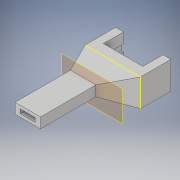
# Autodesk Inventor part: tilt_pillar
Saved by Autodesk Inventor 2018 (Build 220112000, 112)
## iProperties
Created: 2018-04-15
Part Number: tilt_pillar
Material: Generic
Document SubType Name: Modeling
Designer: scwu
Density: 1 g/cm^3
Appearance: Default
Author: scwu
Autodesk Inventor part; units mm, degrees
note: some values were not read from the file. Chosen so that the rebuilt part matches the saved one: second side of "Extrusion5".
ref_plane "YZ Plane" through (0, 0, 0) normal (1, 0, 0) x (0, 1, 0)
ref_plane "XZ Plane" through (0, 0, 0) normal (0, 1, 0) x (-1, 0, 0)
ref_plane "XY Plane" through (0, 0, 0) normal (0, 0, 1) x (1, 0, 0)
sketch "Sketch1" plane through (0, 0, 0) normal (0, 1, 0) x (-1, 0, 0)
  line L0 (-4.4, 0) -> (4.4, 0) construction
  line L1 (0, 0) -> (0, -12) construction
  line L2 (2.65, -12) -> (-2.65, -12) construction
  line L3 (2.65, -12) -> (4.4, 0)
  line L4 (-2.65, -12) -> (-4.4, 0)
  line L5 (0, -12) -> (0, -15.5) construction
  line L6 (0, -15.5) -> (-4, -15.5) construction
  line L7 (0, -15.5) -> (4, -15.5) construction
  line L8 (0, -15.5) -> (4, -15.5) construction
  line L9 (2.65, -12) -> (2.1396, -15.5)
  line L10 (-2.65, -12) -> (-2.1396, -15.5)
  line L11 (2.1396, -15.5) -> (-2.1396, -15.5)
  line L12 (-7.4, 0) -> (12.6, 0) construction
  line L13 (4.4, 0) -> (-4.4, 0)
  dimension "d0" = 8.8
  dimension "d1" = 12
  dimension "d2" = 5.3
  dimension "d3" = 3.5
  dimension "d4" = 4
  dimension "d5" = 4
  dimension "d7" = 3
  constraints: 28 end point, 7 horizontal, 4 collinear, 2 point on line, 2 symmetric about line, 1 midpoint, 1 perpendicular, 1 vertical
  measures "d0" distance of L0.start L0.end
  measures "d1" distance of L1.end L1.start
  measures "d2" distance of L2.start L2.end
  measures "d3" distance of L1.end L5.end
  measures "d4" distance of L5.end L6.end
  measures "d5" distance of L5.end L7.end
  measures "d7" distance of L0.start L12.start
sketch "Sketch2" plane through (0, 0, 0) normal (0, 1, 0) x (-1, 0, 0)
  line L0 (7.4, -46.26) -> (-7.4, -46.26)
  line L1 (-7.4, -46.26) -> (-7.4, 0)
  line L2 (-7.4, 0) -> (7.4, 0)
  line L3 (7.4, 0) -> (7.4, -46.26)
  line L4 (0, 0) -> (0, 4) construction
  line L5 (0, 0) -> (0, -46.26) construction
  dimension "d18" = 4
  dimension "d19" = 50.26
  dimension "d20" = 14.8
  constraints: 12 end point, 2 midpoint, 2 parallel, 2 vertical, 1 horizontal, 1 perpendicular
  measures "d18" distance of L4.start L4.end
  measures "d19" distance of L4.end L5.end
  measures "d20" distance of L1.end L2.end
extrude "Extrusion1" add sketch "Sketch2" along normal mid plane 6
extrude "Extrusion2" cut sketch "Sketch1" along normal mid plane 2.4
sketch "Sketch3" plane through (0, 0, 0) normal (0, 1, 0) x (-1, 0, 0)
  line L0 (0, 0) -> (0, 4) construction
  line L1 (0, 0) -> (0, -46.26) construction
  dimension "d15" = 4
  dimension "d17" = 50.26
  constraints: 4 end point, 2 vertical
  measures "d15" distance of L0.start L0.end
  measures "d17" distance of L0.end L1.end
sketch "Sketch4" plane through (7.4, 3, -46.26) normal (0, 0, -1) x (-1, 0, 0)
  line L0 (-13.95, 5) -> (18.25, 5)
  line L1 (18.25, 5) -> (18.25, -11)
  line L2 (18.25, -11) -> (-13.95, -11)
  line L3 (-13.95, -11) -> (-13.95, 5)
  line L4 (-9.35, 3.1) -> (13.65, 3.1)
  line L5 (13.65, 3.1) -> (13.65, -9.1)
  line L6 (13.65, -9.1) -> (-9.35, -9.1)
  line L7 (-9.35, -9.1) -> (-9.35, 3.1)
  line L8 (2.15, 5) -> (2.15, -11) construction
  line L9 (18.25, -3) -> (-13.95, -3) construction
  line L10 (-9.35, 3.1) -> (-9.35, 5)
  line L11 (13.65, 3.1) -> (13.65, 5)
  line L12 (13.65, -9.1) -> (13.65, -11)
  line L13 (-9.35, -9.1) -> (-9.35, -11)
  circle A0 centre (16.15, -3) radius 1
  circle A1 centre (-11.85, -3) radius 1
  point P0 (7.4, -3)
  point P1 (2.15, -3)
  dimension "d21" = 32.2
  dimension "d22" = 16
  dimension "d23" = 23
  dimension "d24" = 12.2
  dimension "d25" = 2.5
  dimension "d26" = 2
  dimension "d27" = 2.5
  dimension "d28" = 2
  dimension "d43" = 5.25
  constraints: 28 end point, 9 point on line, 5 midpoint, 5 parallel, 2 centre point, 2 coincident, 2 horizontal, 2 perpendicular, 1 horizontal alignment, 2 other
  measures "d21" distance of L1.end L2.end
  measures "d22" distance of L0.end L1.end
  measures "d23" distance of L5.end L6.end
  measures "d24" distance of L4.end L5.end
  measures "d25" distance from line of L5 point (16.15, -3)
  measures "d26" diameter of A0
  measures "d27" distance from line of L7 point (-11.85, -3)
  measures "d28" diameter of A1
  measures "d43" distance of point (7.4, -3) point (2.15, -3)
extrude "Extrusion3" add sketch "Sketch4" along normal blind 15.72 and the other way blind 2 contours L0 L10 L7 L13 L2 L3 | L0 L1 L2 L12 L5 L11
extrude "Extrusion4" add sketch "Sketch4" along normal blind 4 and the other way blind 2 contours L0 L11 L4 L10 | L13 L6 L12 L2
extrude "Extrusion5" add sketch "Sketch4" against normal blind 2 contours A0 | A1
extrude "Extrusion6" add sketch "Sketch4" against normal blind 2 contours L4 L5 L6 L7
sketch "Sketch5" plane through (-10.85, -8, -61.98) normal (-1, 0, 0) x (0, 0, 1)
  line L0 (15.72, 1.9) -> (15.72, 14.1) projected
  line L1 (15.72, 8) -> (6.72, 8) construction
  line L2 (15.72, 6) -> (6.72, 6)
  line L3 (6.72, 6) -> (6.72, 10)
  line L4 (6.72, 10) -> (15.72, 10)
  line L5 (15.72, 10) -> (15.72, 6)
  line L6 (15.72, 6) -> (6.72, 10) construction
  line L7 (6.72, 6) -> (15.72, 10) construction
  point P0 (61.98, 8)
  point P1 (11.22, 8)
  dimension "d44" = 9
  dimension "d45" = 4
  constraints: 14 end point, 4 midpoint, 2 horizontal, 2 parallel, 1 collinear, 1 perpendicular
  measures "d44" distance of L1.start L1.end
  measures "d45" distance of L2.end L3.end
extrude "Extrusion7" cut sketch "Sketch5" against normal blind 6
sketch "Sketch6" plane through (-6.25, -8, -61.98) normal (1, 0, 0) x (0, 0, -1)
  line L0 (-15.72, 10) -> (-6.72, 10) projected
  line L1 (0, 0) -> (0, 16) projected
  line L2 (-6.72, 10) -> (0, 10)
  line L3 (0, 10) -> (0, 6)
  line L4 (0, 6) -> (-6.72, 6)
  line L5 (-6.72, 6) -> (-6.72, 10)
  point P0 (-61.98, 8)
  dimension "d48" = 4
  constraints: 8 end point, 2 parallel, 1 horizontal, 1 perpendicular, 1 point on line
  measures "d48" distance of L2.end L3.end
extrude "Extrusion8" cut sketch "Sketch6" against normal blind 1
ref_plane "Work Plane1" through (7.4, 3, -32.26) normal (0, 0, 1) x (1, 0, 0)
sketch "Sketch7" plane through (7.4, 3, -32.26) normal (0, 0, 1) x (1, 0, 0)
  line L0 (-14.8, 0) -> (0, 0) projected
  line L1 (0, 0) -> (0, -6) projected
  line L2 (0, -6) -> (-14.8, -6) projected
  line L3 (-14.8, 0) -> (-14.8, -6) projected
  point P0 (-7.4, -3)
sketch "Sketch8" plane through (7.4, 3, -44.26) normal (0, 0, 1) x (1, 0, 0)
  line L0 (13.95, 5) -> (-18.25, 5) projected
  line L1 (-18.25, 5) -> (-18.25, -11) projected
  line L2 (-18.25, -11) -> (13.95, -11) projected
  line L3 (13.95, -11) -> (13.95, 5) projected
  point P0 (-7.4, -3)
loft "Loft1" add profiles "Sketch7" section 2 edges at (5.25, 8, -44.26) (-10.85, 0, -44.26) (5.25, -8, -44.26) (21.35, 0, -44.26)
body "Solid1"
